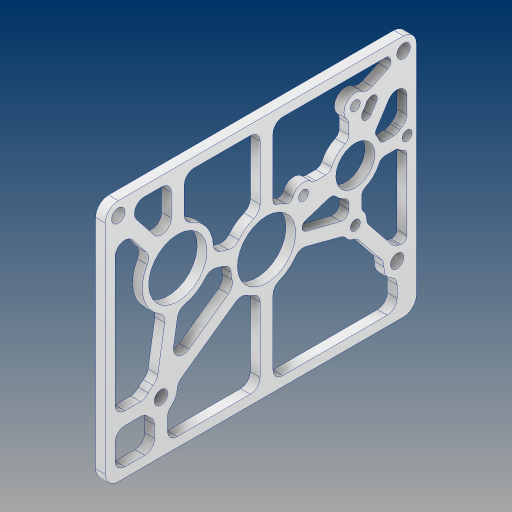
# Autodesk Inventor part: Intake Pivot Gearbox Plate
Saved by Autodesk Inventor 2024.3 (Build 283343000, 343)
## iProperties
Created: 2024-08-02
Part Number: Intake Pivot Gearbox Plate
Material: Aluminum 6061
Document SubType Name: Modeling
Designer: Kenji
Density: 2.7 g/cm^3
Appearance: Aluminum - Flat
Author: Kenji
Autodesk Inventor part; units mm, degrees
ref_plane "YZ Plane" through (0, 0, 0) normal (1, 0, 0) x (0, 1, 0)
ref_plane "XZ Plane" through (0, 0, 0) normal (0, 1, 0) x (-1, 0, 0)
ref_plane "XY Plane" through (0, 0, 0) normal (0, 0, 1) x (1, 0, 0)
sketch "Sketch1" plane through (0, 0, 0) normal (1, 0, 0) x (0, 1, 0)
  line L0 (0, 0) -> (25.4, 0) construction
  line L1 (25.4, 0) -> (25.4, -279.4) construction
  line L2 (25.4, -279.4) -> (0, -279.4) construction
  line L3 (0, -279.4) -> (0, 0) construction
  line L4 (25.4, -279.4) -> (101.6254, -279.4) construction
  line L5 (101.6254, -279.4) -> (101.6254, -38.1) construction
  circle A0 centre (101.6254, -38.1) radius 14.2875 construction
  line L6 (25.4, -19.05) -> (0, -19.05) construction
  line L7 (25.4, -260.35) -> (0, -260.35) construction
  circle A1 centre (101.6254, -38.1) radius 31.115 construction
  line L8 (0, 0) -> (203.2, 0) construction
  line L9 (203.2, 0) -> (203.2, 25.4) construction
  line L10 (203.2, 25.4) -> (0, 25.4) construction
  line L11 (0, 25.4) -> (0, 0) construction
  circle A2 centre (101.6254, -125.1505) radius 30 construction
  circle A3 centre (101.6254, -125.1505) radius 9.525
  circle A4 centre (101.6254, -125.1505) radius 10.16 construction
  circle A5 centre (87.63, -81.6252) radius 35.56 construction
  circle A6 centre (87.63, -81.6252) radius 14.2875
  circle A7 centre (101.6254, -125.1505) radius 25.4 construction
  circle A8 centre (127.0254, -125.1505) radius 2.3876
  circle A9 centre (119.5859, -107.19) radius 2.3876 construction
  circle A10 centre (101.6254, -99.7505) radius 2.3876
  circle A11 centre (83.6649, -107.19) radius 2.3876 construction
  circle A12 centre (76.2254, -125.1505) radius 2.3876
  circle A13 centre (83.6649, -143.111) radius 2.3876 construction
  circle A14 centre (101.6254, -150.5505) radius 2.3876
  circle A15 centre (119.5859, -143.111) radius 2.3876 construction
  circle A16 centre (87.63, -81.6252) radius 11.43 construction
  circle A17 centre (101.6254, -38.1) radius 34.29 construction
  circle A18 centre (101.6254, -38.1) radius 14.2875
  circle A19 centre (101.6254, -38.1) radius 9.525 construction
  circle A20 centre (101.6254, -38.1) radius 35.56 construction
  circle A21 centre (138.4554, -8.89) radius 3.2512
  circle A22 centre (50.8, -29.845) radius 3.2512
  circle A23 centre (87.63, -81.6252) radius 36.83 construction
  line L12 (25.4, -136.1005) -> (57.15, -136.1005) construction
  line L13 (57.15, -136.1005) -> (57.15, -155.1505) construction
  line L14 (57.15, -155.1505) -> (25.4, -155.1505) construction
  line L15 (25.4, -155.1505) -> (25.4, -136.1005) construction
  circle A24 centre (50.8, -145.6255) radius 3.2512
  circle A25 centre (138.4554, -148.8005) radius 3.2512
  circle A26 centre (138.4554, -148.8005) radius 6.35 construction
  line L16 (31.75, -155.1505) -> (138.4554, -155.1505)
  circle A27 centre (138.4554, -8.89) radius 6.35 construction
  line L17 (144.8054, -8.89) -> (144.8054, -148.8005)
  line L18 (25.4, -148.8005) -> (25.4, -8.89)
  line L19 (31.75, -2.54) -> (138.4554, -2.54)
  arc A28 (138.4554, -155.1505) -> (144.8054, -148.8005) centre (138.4554, -148.8005) ccw
  arc A29 (144.8054, -8.89) -> (138.4554, -2.54) centre (138.4554, -8.89) ccw
  arc A30 (31.75, -2.54) -> (25.4, -8.89) centre (31.75, -8.89) ccw
  arc A31 (25.4, -148.8005) -> (31.75, -155.1505) centre (31.75, -148.8005) ccw
  circle A32 centre (87.63, -81.6252) radius 15.5575 construction
  line L20 (25.4, -39.37) -> (57.15, -39.37) construction
  line L21 (57.15, -39.37) -> (57.15, -20.32) construction
  line L22 (25.4, -20.32) -> (25.4, -39.37) construction
  line L23 (57.15, -20.32) -> (25.4, -20.32) construction
  point P0 (50.8, -81.6252)
  point P1 (57.15, -145.6255)
  point P2 (25.4, -2.54)
  dimension "d30" = 50.8
  dimension "d0" = 25.4
  dimension "d1" = 279.4
  dimension "d2" = 76.2254
  dimension "d3" = 241.3
  dimension "d4" = 28.575
  dimension "d5" = 19.05
  dimension "d6" = 19.05
  dimension "d7" = 62.23
  dimension "d8" = 25.4
  dimension "d9" = 203.2
  dimension "d11" = 60
  dimension "d20" = 19.05
  dimension "d27" = 20.32
  dimension "d28" = 71.12
  dimension "d29" = 28.575
  dimension "d31" = 4.7752
  dimension "d34" = 360
  dimension "d36" = 22.86
  dimension "d37" = 68.58
  dimension "d38" = 28.575
  dimension "d39" = 19.05
  dimension "d40" = 1.27
  dimension "d41" = 6.5024
  dimension "d44" = 6.5024
  dimension "d47" = 1.27
  dimension "d48" = 25.4
  dimension "d49" = 31.75
  dimension "d50" = 19.05
  dimension "d51" = 6.5024
  dimension "d52" = 6.35
  dimension "d53" = 9.525
  dimension "d56" = 6.5024
  dimension "d57" = 12.7
  dimension "d58" = 12.7
  dimension "d62" = 6.35
  dimension "d185" = 31.115
  dimension "d188" = 31.75
  dimension "d189" = 19.05
  dimension "d192" = 36.83
  dimension "d193" = 9.525
  dimension "d194" = 1.27
  constraints: 48 end point, 31 centre point, 13 tangent, 12 coincident, 12 point on circle, 12 point on line, 7 parallel, 7 perpendicular, 6 horizontal, 4 horizontal alignment, 3 vertical alignment, 2 equal radius, 1 concentric, 1 midpoint, 1 vertical, 21 other
  measures "d0" distance of L1.end L2.end
  measures "d1" distance of L0.end L1.end
  measures "d2" distance of L1.end L4.end
  measures "d3" distance of L4.end L5.end
  measures "d4" diameter of A0
  measures "d5" distance between parallel lines of L0 L6
  measures "d6" distance between parallel lines of L7 L2
  measures "d7" diameter of A1
  measures "d8" distance of L9.end L8.end
  measures "d9" distance between parallel lines of L11 L9
  measures "d11" diameter of A2
  measures "d20" diameter of A3
  measures "d27" diameter of A4
  measures "d28" diameter of A5
  measures "d29" diameter of A6
  measures "d31" diameter of A8
  measures "d36" diameter of A16
  measures "d37" diameter of A17
  measures "d38" diameter of A18
  measures "d39" diameter of A19
  measures "d40" radial gap between concentric circles of A17 A20
  measures "d41" diameter of A21
  measures "d44" diameter of A22
  measures "d48" distance from line of L1 point (50.8, -81.625)
  measures "d49" distance of L13.end L14.end
  measures "d50" distance of L12.end L13.end
  measures "d51" diameter of A24
  measures "d52" distance of point (57.15, -145.625) A24.centre
  measures "d53" distance from line of L12 A24.centre
  measures "d56" diameter of A25
  measures "d57" diameter of A26
  measures "d58" diameter of A27
  measures "d62" radius of A30
  measures "d185" diameter of A32
  measures "d188" distance of L22.start L21.end
  measures "d189" distance of L21.end L20.end
  measures "d192" horizontal distance of L5.end A29.centre
  measures "d193" distance from line of L20 A22.centre
  measures "d194" distance between parallel lines of L23 L6
extrude "Extrusion1" add sketch "Sketch1" along normal blind 4.7625
sketch "Sketch2" plane through (0, 0, 0) normal (-1, 0, 0) x (0, 0, 1)
  line L0 (-155.1505, 31.75) -> (-155.1505, 138.4554) projected
  arc A0 (-155.1505, 31.75) -> (-148.8005, 25.4) centre (-148.8005, 31.75) ccw projected
  line L1 (-8.89, 25.4) -> (-148.8005, 25.4) projected
  arc A1 (-8.89, 25.4) -> (-2.54, 31.75) centre (-8.89, 31.75) ccw projected
  line L2 (-2.54, 138.4554) -> (-2.54, 31.75) projected
  arc A2 (-2.54, 138.4554) -> (-8.89, 144.8054) centre (-8.89, 138.4554) ccw projected
  line L3 (-148.8005, 144.8054) -> (-8.89, 144.8054) projected
  arc A3 (-148.8005, 144.8054) -> (-155.1505, 138.4554) centre (-148.8005, 138.4554) ccw projected
  circle A4 centre (-125.1505, 101.6254) radius 9.525 projected
  circle A5 centre (-125.1505, 127.0254) radius 2.3876 projected
  circle A6 centre (-125.1505, 76.2254) radius 2.3876 projected
  circle A7 centre (-150.5505, 101.6254) radius 2.3876 projected
  circle A8 centre (-38.1, 101.6254) radius 14.2875 projected
  circle A9 centre (-29.845, 50.8) radius 3.2512 projected
  circle A10 centre (-145.6255, 50.8) radius 3.2512 projected
  circle A11 centre (-148.8005, 138.4554) radius 3.2512 projected
  circle A12 centre (-8.89, 138.4554) radius 3.2512 projected
  circle A13 centre (-99.7505, 101.6254) radius 2.3876 projected
  circle A14 centre (-81.6252, 87.63) radius 14.2875 projected
  arc A15 (-7.3152, 138.4554) -> (-8.89, 140.0302) centre (-8.89, 138.4554) ccw construction
  line L4 (-7.3152, 138.4554) -> (-7.3152, 31.75) construction
  arc A16 (-8.89, 30.1752) -> (-7.3152, 31.75) centre (-8.89, 31.75) ccw construction
  line L5 (-8.89, 30.1752) -> (-148.8005, 30.1752) construction
  arc A17 (-150.3753, 31.75) -> (-148.8005, 30.1752) centre (-148.8005, 31.75) ccw construction
  line L6 (-150.3753, 31.75) -> (-150.3753, 96.0656) construction
  arc A18 (-148.8005, 140.0302) -> (-150.3753, 138.4554) centre (-148.8005, 138.4554) ccw construction
  line L7 (-148.8005, 140.0302) -> (-8.89, 140.0302) construction
  circle A19 centre (-81.6252, 87.63) radius 17.4625 construction
  circle A20 centre (-38.1, 101.6254) radius 17.4625 construction
  circle A21 centre (-99.7505, 101.6254) radius 5.5626 construction
  circle A22 centre (-125.1505, 76.2254) radius 5.5626 construction
  circle A23 centre (-145.6255, 50.8) radius 6.4262 construction
  circle A24 centre (-150.5505, 101.6254) radius 5.5626 construction
  circle A25 centre (-148.8005, 138.4554) radius 6.4262 construction
  circle A26 centre (-125.1505, 127.0254) radius 5.5626 construction
  circle A27 centre (-8.89, 138.4554) radius 6.4262 construction
  line L8 (-27.2489, 115.3072) -> (-12.8832, 133.4205) construction
  line L9 (-38.1, 119.0879) -> (-38.1, 140.0302) construction
  line L10 (-81.6252, 105.0925) -> (-81.6252, 140.0302) construction
  line L11 (-81.6252, 70.1675) -> (-81.6252, 30.1752) construction
  line L12 (-98.2495, 92.9755) -> (-113.0601, 97.7378) construction
  line L13 (-125.1505, 88.9254) -> (-125.1505, 81.788) construction
  line L14 (-137.8505, 101.6254) -> (-144.9879, 101.6254) construction
  line L15 (-125.1505, 114.3254) -> (-125.1505, 121.4628) construction
  line L16 (-130.1588, 129.4459) -> (-143.0146, 135.6591) construction
  line L17 (-132.0127, 112.3119) -> (-145.3282, 133.0481) construction
  line L18 (-128.6394, 71.893) -> (-141.5949, 55.8051) construction
  line L19 (-119.7695, 77.6353) -> (-98.5175, 83.2038) construction
  line L20 (-65.001, 92.9755) -> (-54.7242, 96.2799) construction
  line L21 (-105.3131, 101.6254) -> (-112.4505, 101.6254) construction
  line L22 (-105.7524, 104.8004) -> (-110.6008, 104.8004)
  line L23 (-84.8002, 106.68) -> (-84.8002, 135.255)
  line L24 (-121.9755, 116.1751) -> (-121.9755, 121.0235)
  arc A28 (-121.1079, 123.2044) -> (-128.4744, 131.4857) centre (-125.1505, 127.0254) ccw
  arc A29 (-86.5147, 104.394) -> (-91.0129, 102.3545) centre (-81.6252, 87.63) ccw
  arc A30 (-94.5285, 103.5419) -> (-103.5715, 105.668) centre (-99.7505, 101.6254) ccw
  line L25 (-140.0243, 140.0302) -> (-89.5754, 140.0302)
  arc A31 (-84.8002, 135.255) -> (-89.5754, 140.0302) centre (-89.5754, 135.255) ccw
  circle A32 centre (-92.293, 104.3624) radius 2.3812 construction
  circle A33 centre (-87.1815, 106.68) radius 2.3813 construction
  arc A34 (-94.5285, 103.5419) -> (-91.0129, 102.3545) centre (-92.293, 104.3624) ccw
  arc A35 (-86.5147, 104.394) -> (-84.8002, 106.68) centre (-87.1815, 106.68) ccw
  line L26 (-130.6445, 126.1543) -> (-140.0459, 130.698) construction
  line L27 (-128.3255, 112.4458) -> (-140.0459, 130.698) construction
  line L28 (-128.3255, 112.4458) -> (-128.3255, 122.4579) construction
  arc A36 (-130.6445, 126.1543) -> (-128.3255, 122.4579) centre (-125.1505, 127.0254) ccw construction
  circle A37 centre (-133.4624, 124.8644) radius 2.3876 construction
  circle A38 centre (-132.6851, 124.4887) radius 2.3876 construction
  arc A39 (-132.4235, 127.0141) -> (-135.4715, 123.5743) centre (-133.4624, 124.8644) ccw
  line L29 (-132.4235, 127.0141) -> (-131.6462, 126.6384)
  arc A40 (-130.4223, 125.2505) -> (-131.6462, 126.6384) centre (-132.6851, 124.4887) ccw
  arc A41 (-130.4223, 125.2505) -> (-129.1931, 123.2044) centre (-125.1505, 127.0254) ccw
  line L30 (-128.3255, 121.0235) -> (-128.3255, 112.4458) construction
  line L31 (-135.4715, 123.5743) -> (-128.3255, 112.4458) construction
  line L32 (-135.4001, 111.711) -> (-141.582, 121.338)
  line L33 (-139.1752, 104.8004) -> (-143.9426, 104.8004)
  arc A42 (-146.9949, 105.9033) -> (-147.8868, 106.5087) centre (-150.5505, 101.6254) ccw
  line L34 (-150.3753, 118.7578) -> (-150.3753, 110.7008)
  arc A43 (-150.3753, 110.7008) -> (-147.8868, 106.5087) centre (-145.6001, 110.7008) ccw
  line L35 (-139.7002, 98.4504) -> (-144.5486, 98.4504)
  line L36 (-131.7679, 73.0702) -> (-143.1491, 58.9372)
  line L37 (-128.3255, 87.0757) -> (-128.3255, 82.2273)
  arc A44 (-129.1931, 80.0464) -> (-130.7124, 76.1392) centre (-125.1505, 76.2254) ccw
  line L38 (-150.3753, 50.8) -> (-152.0517, 50.8) construction
  line L39 (-150.3753, 53.975) -> (-151.2126, 53.975) construction
  arc A45 (-146.3385, 57.1865) -> (-147.3478, 56.9911) centre (-145.6255, 50.8) ccw
  line L40 (-150.3753, 59.2914) -> (-150.3753, 93.5556)
  arc A46 (-131.7679, 73.0702) -> (-130.7124, 76.1392) centre (-135.4871, 76.0652) ccw
  arc A47 (-146.3385, 57.1865) -> (-143.1491, 58.9372) centre (-146.8683, 61.9322) ccw
  circle A48 centre (-147.9877, 59.2914) radius 2.3876 construction
  arc A49 (-150.3753, 59.2914) -> (-147.3478, 56.9911) centre (-147.9877, 59.2914) ccw
  line L41 (-121.5369, 80.4544) -> (-99.0407, 86.3489) construction
  line L42 (-121.9755, 87.0757) -> (-121.9755, 84.4536)
  circle A50 centre (-101.4677, 88.1812) radius 2.3876 construction
  line L43 (-100.8625, 85.8716) -> (-117.9957, 81.3823)
  line L44 (-112.2712, 94.149) -> (-100.981, 90.5187)
  arc A51 (-99.081, 88.1149) -> (-100.981, 90.5187) centre (-101.4677, 88.1812) ccw
  arc A52 (-100.8625, 85.8716) -> (-99.081, 88.1149) centre (-101.4677, 88.1812) ccw
  line L45 (-117.9536, 74.829) -> (-100.9103, 79.2947)
  line L46 (-126.8222, 69.0874) -> (-138.2034, 54.9544)
  line L47 (-84.8002, 66.862) -> (-84.8002, 34.9504)
  arc A53 (-95.8187, 77.4572) -> (-87.8683, 71.3216) centre (-81.6252, 87.63) ccw
  arc A54 (-124.0488, 70.773) -> (-120.6267, 72.9885) centre (-125.1505, 76.2254) ccw
  arc A55 (-142.886, 44.987) -> (-139.2338, 51.4651) centre (-145.6255, 50.8) ccw
  line L48 (-150.3753, 47.625) -> (-151.2126, 47.625) construction
  arc A56 (-138.2034, 54.9544) -> (-139.2338, 51.4651) centre (-134.4843, 51.9594) ccw
  arc A57 (-117.9536, 74.829) -> (-120.6267, 72.9885) centre (-116.7433, 70.2097) ccw
  arc A58 (-124.0488, 70.773) -> (-126.8222, 69.0874) centre (-123.103, 66.0924) ccw
  arc A59 (-95.8187, 77.4572) -> (-100.9103, 79.2947) centre (-99.6999, 74.6754) ccw
  arc A60 (-84.8002, 66.862) -> (-87.8683, 71.3216) centre (-89.5754, 66.862) ccw
  arc A61 (-89.5754, 30.1752) -> (-84.8002, 34.9504) centre (-89.5754, 34.9504) ccw
  line L49 (-145.6255, 40.6674) -> (-145.6255, 34.9504)
  line L50 (-89.5754, 30.1752) -> (-140.8503, 30.1752)
  arc A62 (-142.886, 44.987) -> (-145.6255, 40.6674) centre (-140.8503, 40.6674) ccw
  arc A63 (-145.6255, 34.9504) -> (-140.8503, 30.1752) centre (-140.8503, 34.9504) ccw
  line L51 (-78.4502, 108.398) -> (-78.4502, 135.255)
  line L52 (-62.8261, 97.0099) -> (-58.8429, 98.2907)
  line L53 (-41.275, 122.3934) -> (-41.275, 135.255)
  arc A64 (-68.0108, 98.5655) -> (-75.3822, 103.9384) centre (-81.6252, 87.63) ccw
  arc A65 (-44.343, 117.9338) -> (-55.5366, 102.5765) centre (-38.1, 101.6254) ccw
  line L54 (-73.675, 140.0302) -> (-46.0502, 140.0302)
  arc A66 (-73.675, 140.0302) -> (-78.4502, 135.255) centre (-73.675, 135.255) ccw
  arc A67 (-41.275, 135.255) -> (-46.0502, 140.0302) centre (-46.0502, 135.255) ccw
  arc A68 (-44.343, 117.9338) -> (-41.275, 122.3934) centre (-46.0502, 122.3934) ccw
  arc A69 (-58.8429, 98.2907) -> (-55.5366, 102.5765) centre (-60.3047, 102.8366) ccw
  arc A70 (-68.0108, 98.5655) -> (-62.8261, 97.0099) centre (-64.2878, 101.5559) ccw
  arc A71 (-78.4502, 108.398) -> (-75.3822, 103.9384) centre (-73.675, 108.398) ccw
  line L55 (-60.8823, 90.9647) -> (-56.8991, 92.2455)
  line L56 (-78.4502, 66.862) -> (-78.4502, 34.9504)
  line L57 (-73.675, 30.1752) -> (-37.7952, 30.1752)
  arc A72 (-64.7171, 83.2648) -> (-64.1887, 86.6789) centre (-81.6252, 87.63) ccw
  arc A73 (-60.8823, 90.9647) -> (-64.1887, 86.6789) centre (-59.4206, 86.4188) ccw
  arc A74 (-75.3822, 71.3216) -> (-78.4502, 66.862) centre (-73.675, 66.862) ccw
  arc A75 (-78.4502, 34.9504) -> (-73.675, 30.1752) centre (-73.675, 34.9504) ccw
  arc A76 (-51.7145, 90.6899) -> (-41.6477, 84.5271) centre (-38.1, 101.6254) ccw
  arc A77 (-51.7145, 90.6899) -> (-56.8991, 92.2455) centre (-55.4374, 87.6995) ccw
  line L58 (-34.925, 124.4437) -> (-34.925, 135.255)
  line L59 (-26.4084, 121.4764) -> (-17.834, 132.2877)
  line L60 (-21.5753, 140.0302) -> (-30.1498, 140.0302)
  arc A78 (-15.1203, 140.0302) -> (-7.3152, 132.2251) centre (-8.89, 138.4554) ccw construction
  arc A79 (-17.834, 132.2877) -> (-21.5753, 140.0302) centre (-21.5753, 135.255) ccw
  arc A80 (-30.1498, 140.0302) -> (-34.925, 135.255) centre (-30.1498, 135.255) ccw
  arc A81 (-29.3232, 86.5288) -> (-23.0747, 110.5236) centre (-38.1, 101.6254) ccw
  arc A82 (-22.7073, 115.9241) -> (-23.0747, 110.5236) centre (-18.9659, 112.9569) ccw
  arc A83 (-142.4734, 137.331) -> (-142.4017, 137.8628) centre (-148.8005, 138.4554) ccw
  arc A84 (-150.3753, 132.2251) -> (-148.4532, 132.0386) centre (-148.8005, 138.4554) ccw construction
  arc A85 (-141.582, 121.338) -> (-150.3753, 118.7578) centre (-145.6001, 118.7578) ccw
  circle A86 centre (-140.0243, 137.6426) radius 2.3876 construction
  circle A87 centre (-140.1227, 136.9132) radius 2.3876 construction
  line L61 (-133.4058, 131.0152) -> (-141.1616, 134.7635)
  arc A88 (-140.0243, 140.0302) -> (-142.4017, 137.8628) centre (-140.0243, 137.6426) ccw
  arc A89 (-142.4734, 137.331) -> (-141.1616, 134.7635) centre (-140.1227, 136.9132) ccw
  arc A90 (-133.4058, 131.0152) -> (-128.4744, 131.4857) centre (-131.3279, 135.3146) ccw
  circle A91 centre (-125.1505, 101.6254) radius 12.7 construction
  circle A92 centre (-130.7131, 120.5828) radius 2.3876 construction
  arc A93 (-128.3255, 121.0235) -> (-129.1931, 123.2044) centre (-131.5005, 121.0235) ccw
  line L62 (-128.3255, 121.0235) -> (-128.3255, 120.5828)
  arc A94 (-132.7221, 119.2927) -> (-128.3255, 120.5828) centre (-130.7131, 120.5828) ccw
  line L63 (-132.7221, 119.2927) -> (-135.4715, 123.5743)
  arc A95 (-113.5108, 106.7054) -> (-120.0705, 113.2651) centre (-125.1505, 101.6254) ccw
  arc A96 (-121.9755, 116.1751) -> (-120.0705, 113.2651) centre (-118.8005, 116.1751) ccw
  arc A97 (-113.5108, 106.7054) -> (-110.6008, 104.8004) centre (-110.6008, 107.9754) ccw
  arc A98 (-105.7524, 104.8004) -> (-103.5715, 105.668) centre (-105.7524, 107.9754) ccw
  arc A99 (-135.4692, 109.029) -> (-136.9558, 106.3077) centre (-125.1505, 101.6254) ccw
  circle A100 centre (-137.4092, 110.4209) radius 2.3876 construction
  circle A101 centre (-139.1752, 107.188) radius 2.3876 construction
  arc A102 (-135.4692, 109.029) -> (-135.4001, 111.711) centre (-137.4092, 110.4209) ccw
  arc A103 (-139.1752, 104.8004) -> (-136.9558, 106.3077) centre (-139.1752, 107.188) ccw
  arc A104 (-121.9755, 84.4536) -> (-117.9957, 81.3823) centre (-118.8005, 84.4536) ccw
  arc A105 (-120.0705, 89.9857) -> (-115.6246, 93.2262) centre (-125.1505, 101.6254) ccw
  arc A106 (-112.2712, 94.149) -> (-115.6246, 93.2262) centre (-113.2431, 91.1264) ccw
  arc A107 (-120.0705, 89.9857) -> (-121.9755, 87.0757) centre (-118.8005, 87.0757) ccw
  arc A108 (-148.4177, 96.4879) -> (-146.7295, 97.5828) centre (-150.5505, 101.6254) ccw
  arc A109 (-136.7902, 96.5454) -> (-130.2305, 89.9857) centre (-125.1505, 101.6254) ccw
  arc A110 (-136.7902, 96.5454) -> (-139.7002, 98.4504) centre (-139.7002, 95.2754) ccw
  arc A111 (-128.3255, 87.0757) -> (-130.2305, 89.9857) centre (-131.5005, 87.0757) ccw
  arc A112 (-129.1931, 80.0464) -> (-128.3255, 82.2273) centre (-131.5005, 82.2273) ccw
  arc A113 (-144.5486, 98.4504) -> (-146.7295, 97.5828) centre (-144.5486, 95.2754) ccw
  arc A114 (-148.4177, 96.4879) -> (-150.3753, 93.5556) centre (-147.2003, 93.5556) ccw
  arc A115 (-121.1079, 123.2044) -> (-121.9755, 121.0235) centre (-118.8005, 121.0235) ccw
  arc A116 (-146.9949, 105.9033) -> (-143.9426, 104.8004) centre (-143.9426, 109.5756) ccw
  line L64 (-22.7073, 115.9241) -> (-15.8318, 124.5933)
  line L65 (-35.3004, 84.3888) -> (-30.3662, 54.0091) construction
  line L66 (-29.845, 47.5488) -> (-29.845, 30.1752) construction
  line L67 (-32.4944, 52.6844) -> (-67.3952, 77.5085) construction
  circle A117 centre (-29.845, 50.8) radius 3.2512 projected
  circle A118 centre (-29.845, 50.8) radius 8.0264 construction
  line L68 (-39.8617, 54.0284) -> (-66.5418, 73.0053)
  line L69 (-31.6366, 81.635) -> (-28.3197, 61.2129)
  line L70 (-37.9044, 80.617) -> (-36.0295, 69.0731)
  line L71 (-43.5107, 64.4163) -> (-62.8613, 78.1799)
  arc A119 (-64.7171, 83.2648) -> (-62.8613, 78.1799) centre (-60.0935, 82.0712) ccw
  arc A120 (-75.3822, 71.3216) -> (-71.9542, 73.0901) centre (-81.6252, 87.63) ccw
  arc A121 (-37.9044, 80.617) -> (-41.6477, 84.5271) centre (-42.6179, 79.8515) ccw
  arc A122 (-43.5107, 64.4163) -> (-36.0295, 69.0731) centre (-40.7429, 68.3076) ccw
  arc A123 (-66.5418, 73.0053) -> (-71.9542, 73.0901) centre (-69.3096, 69.1141) ccw
  line L72 (-33.02, 40.7663) -> (-33.02, 34.9504)
  line L73 (-26.67, 40.7663) -> (-26.67, 34.9504)
  arc A124 (-37.8606, 50.3844) -> (-34.8296, 44.509) centre (-29.845, 50.8) ccw
  arc A125 (-37.8606, 50.3844) -> (-39.8617, 54.0284) centre (-42.6294, 50.1371) ccw
  arc A126 (-33.02, 40.7663) -> (-34.8296, 44.509) centre (-37.7952, 40.7663) ccw
  arc A127 (-37.7952, 30.1752) -> (-33.02, 34.9504) centre (-37.7952, 34.9504) ccw
  arc A128 (-29.3232, 86.5288) -> (-31.6366, 81.635) centre (-26.9231, 82.4006) ccw
  arc A129 (-28.3197, 61.2129) -> (-25.9334, 57.8087) centre (-23.6062, 61.9785) ccw
  arc A130 (-24.8604, 44.509) -> (-26.67, 40.7663) centre (-21.8948, 40.7663) ccw
  arc A131 (-26.67, 34.9504) -> (-21.8948, 30.1752) centre (-21.8948, 34.9504) ccw
  arc A132 (-7.3152, 121.626) -> (-15.8318, 124.5933) centre (-12.0904, 121.626) ccw
  line L74 (-21.8186, 50.8) -> (-7.3152, 50.8) construction
  line L75 (-19.8113, 53.975) -> (-12.0904, 53.975)
  line L76 (-19.8113, 47.625) -> (-12.0904, 47.625)
  arc A133 (-23.554, 55.7846) -> (-25.9334, 57.8087) centre (-29.845, 50.8) ccw
  arc A134 (-24.8604, 44.509) -> (-23.554, 45.8154) centre (-29.845, 50.8) ccw
  line L77 (-7.3152, 58.7502) -> (-7.3152, 121.626)
  arc A135 (-7.3152, 42.8498) -> (-12.0904, 47.625) centre (-12.0904, 42.8498) ccw
  arc A136 (-19.8113, 47.625) -> (-23.554, 45.8154) centre (-19.8113, 42.8498) ccw
  line L78 (-21.8948, 30.1752) -> (-12.0904, 30.1752)
  line L79 (-7.3152, 42.8498) -> (-7.3152, 34.9504)
  arc A137 (-12.0904, 30.1752) -> (-7.3152, 34.9504) centre (-12.0904, 34.9504) ccw
  arc A138 (-23.554, 55.7846) -> (-19.8113, 53.975) centre (-19.8113, 58.7502) ccw
  arc A139 (-12.0904, 53.975) -> (-7.3152, 58.7502) centre (-12.0904, 58.7502) ccw
  arc A140 (-34.925, 124.4437) -> (-26.4084, 121.4764) centre (-30.1498, 124.4437) ccw
  point P0 (0, 0)
  point P1 (-84.8002, 140.0302)
  point P2 (-121.9755, 122.4579)
  point P3 (-121.9755, 113.9221)
  point P4 (-104.318, 104.8004)
  point P5 (-112.8538, 104.8004)
  point P6 (-148.4532, 132.0386)
  point P7 (-145.983, 104.8004)
  point P8 (-150.3753, 107.1852)
  point P9 (-130.4881, 74.6594)
  point P10 (-144.5941, 57.1429)
  point P11 (-128.3255, 80.7929)
  point P12 (-128.3255, 89.3287)
  point P13 (-145.983, 98.4504)
  point P14 (-137.4472, 98.4504)
  point P15 (-121.9755, 89.3287)
  point P16 (-121.9755, 80.7929)
  point P17 (-119.9274, 74.3118)
  point P18 (-97.4312, 80.2063)
  point P19 (-125.5424, 70.6766)
  point P20 (-139.6484, 53.1601)
  point P21 (-84.8002, 70.4586)
  point P22 (-84.8002, 30.1752)
  point P23 (-145.6255, 44.3738)
  point P24 (-145.6255, 30.1752)
  point P25 (-78.4502, 104.8014)
  point P26 (-78.4502, 140.0302)
  point P27 (-66.25, 95.909)
  point P28 (-55.419, 99.3916)
  point P29 (-41.275, 118.7968)
  point P30 (-41.275, 140.0302)
  point P31 (-64.3062, 89.8638)
  point P32 (-53.4752, 93.3464)
  point P33 (-78.4502, 70.4586)
  point P34 (-78.4502, 30.1752)
  point P35 (-8.89, 30.1752)
  point P36 (-53.4752, 93.3464)
  point P37 (-34.925, 118.7968)
  point P38 (-29.9174, 117.0521)
  point P39 (-14.8494, 136.0509)
  point P40 (-34.925, 118.7968)
  point P41 (-29.9174, 117.0521)
  point P42 (-142.4734, 137.331)
  point P43 (-99.0812, 88.1088)
  point P44 (-9.8742, 132.105)
  point P45 (-37.6924, 52.4855)
  point P46 (-69.4726, 75.0899)
  point P47 (-32.2132, 85.1851)
  point P48 (-27.8929, 58.5854)
  point P49 (-38.481, 84.1671)
  point P50 (-65.7921, 80.2645)
  point P51 (-33.02, 43.4283)
  point P52 (-33.02, 30.1752)
  point P53 (-26.67, 43.4283)
  point P54 (-26.67, 30.1752)
  point P55 (-22.4733, 53.975)
  point P56 (-7.3152, 53.975)
  point P57 (-22.4733, 47.625)
  point P58 (-7.3152, 47.625)
  point P59 (-7.3152, 30.1752)
  dimension "d65" = 3.175
  dimension "d66" = 3.175
  dimension "d68" = 3.175
  dimension "d69" = 3.175
  dimension "d70" = 3.175
  dimension "d71" = 3.175
  dimension "d72" = 3.175
  dimension "d73" = 3.175
  dimension "d75" = 3.175
  dimension "d76" = 3.175
  dimension "d78" = 3.175
  dimension "d79" = 3.175
  dimension "d84" = 4.7752
  dimension "d85" = 4.7625
  dimension "d86" = 4.7625
  dimension "d89" = 3.175
  dimension "d90" = 3.175
  dimension "d91" = 3.175
  dimension "d92" = 4.7752
  dimension "d95" = 4.7752
  dimension "d98" = 3.175
  dimension "d99" = 3.175
  dimension "d103" = 4.7752
  dimension "d105" = 3.175
  dimension "d106" = 3.175
  dimension "d107" = 3.175
  dimension "d108" = 3.175
  dimension "d110" = 4.7752
  dimension "d113" = 4.7752
  dimension "d116" = 3.175
  dimension "d117" = 3.175
  dimension "d122" = 4.7752
  dimension "d123" = 3.175
  dimension "d124" = 3.175
  dimension "d125" = 3.175
  dimension "d126" = 3.175
  dimension "d128" = 4.7752
  dimension "d129" = 4.7752
  dimension "d130" = 4.7752
  dimension "d131" = 4.7752
  dimension "d132" = 3.175
  dimension "d133" = 3.175
  dimension "d134" = 3.175
  dimension "d135" = 4.7752
  dimension "d136" = 4.7752
  dimension "d137" = 3.175
  dimension "d139" = 3.175
  dimension "d142" = 4.7752
  dimension "d145" = 4.7752
  dimension "d148" = 3.175
  dimension "d149" = 3.175
  dimension "d150" = 4.7752
  dimension "d151" = 4.7752
  dimension "d157" = 4.7752
  dimension "d161" = 4.7752
  dimension "d163" = 4.7752
  dimension "d164" = 4.7752
  dimension "d165" = 4.7752
  dimension "d166" = 4.7752
  dimension "d169" = 3.175
  dimension "d172" = 4.7752
  dimension "d173" = 3.175
  dimension "d174" = 3.175
  dimension "d175" = 3.175
  constraints: 290 point on circle, 151 end point, 143 tangent, 126 point on line, 118 centre point, 36 parallel, 24 equal radius, 18 concentric, 7 collinear, 4 horizontal, 4 vertical, 2 perpendicular, 141 other
  measures "d68" radial gap between concentric circles of A13 A21
  measures "d71" radial gap between concentric circles of A7 A24
  measures "d73" radial gap between concentric circles of A5 A26
  measures "d75" radial gap between concentric circles of A12 A27
  measures "d76" distance between parallel lines of L21 L22
  measures "d78" distance between parallel lines of L10 L23
  measures "d79" distance between parallel lines of L15 L24
  measures "d84" radius of A31
  measures "d85" diameter of A32
  measures "d86" diameter of A33
  measures "d89" distance between parallel lines of L16 L26
  measures "d90" distance between parallel lines of L17 L27
  measures "d91" distance between parallel lines of L15 L28
  measures "d92" diameter of A37
  measures "d95" diameter of A38
  measures "d98" distance between parallel lines of L17 L32
  measures "d99" distance between parallel lines of L14 L33
  measures "d103" radius of A43
  measures "d105" distance between parallel lines of L14 L35
  measures "d106" distance between parallel lines of L18 L36
  measures "d107" distance between parallel lines of L13 L37
  measures "d108" distance between parallel lines of L38 L39
  measures "d110" radius of A46
  measures "d113" diameter of A48
  measures "d116" distance between parallel lines of L19 L41
  measures "d117" distance between parallel lines of L13 L42
  measures "d122" diameter of A50
  measures "d123" distance between parallel lines of L19 L45
  measures "d124" distance between parallel lines of L18 L46
  measures "d125" distance between parallel lines of L11 L47
  measures "d126" distance between parallel lines of L38 L48
  measures "d128" radius of A56
  measures "d129" radius of A57
  measures "d130" radius of A61
  measures "d131" radius of A62
  measures "d132" distance between parallel lines of L10 L51
  measures "d133" distance between parallel lines of L20 L52
  measures "d134" distance between parallel lines of L9 L53
  measures "d135" radius of A66
  measures "d136" radius of A71
  measures "d137" distance between parallel lines of L20 L55
  measures "d139" distance between parallel lines of L11 L56
  measures "d142" radius of A73
  measures "d145" radius of A77
  measures "d148" distance between parallel lines of L9 L58
  measures "d149" distance between parallel lines of L8 L59
  measures "d150" radius of A79
  measures "d151" radius of A80
  measures "d157" radius of A82
  measures "d161" distance between parallel lines of L7 L3
  measures "d163" radius of A85
  measures "d164" diameter of A86
  measures "d165" diameter of A87
  measures "d166" radius of A90
  measures "d172" diameter of A92
  measures "d173" radius of A93
  measures "d174" radius of A96
  measures "d175" radius of A98
extrude "Extrusion4" cut sketch "Sketch2" against normal blind 25.4 contours L22 A97 A95 A96 L24 A115 A28 A90 L61 A89 A83 A88 L25 A31 L23 A35 A29 A34 A30 A98 | L29 A40 A41 A93 L62 A94 L63 A39 | A102 A99 A103 L33 A116 A42 A43 L34 A85 L32 | A110 A109 A111 L37 A112 A44 A46 L36 A47 A45 A49 L40 A114 A108 A113 L35 | A107 A105 A106 L44 A51 A52 L43 A104 L42 | L45 A59 A53 A60 L47 A61 L50 A63 L49 A62 A55 A56 L46 A58 A54 A57 | L51 A66 L54 A67 L53 A68 A65 A69 L52 A70 A64 A71
extrude "Extrusion5" cut sketch "Sketch2" against normal blind 4.7625 contours L55 A77 A76 A121 L70 A122 L71 A119 A72 A73 | A74 A120 A123 L68 A125 A124 A126 L72 A127 L57 A75 L56 | L58 A80 L60 A79 L59 A140 | A81 A82 L64 A132 L77 A139 L75 A138 A133 A129 L69 A128 | A130 A134 A136 L76 A135 L79 A137 L78 A131 L73
body "Solid1"
